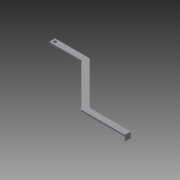
# Autodesk Inventor part: Z-PickupArm
Saved by Autodesk Inventor 2013 (Build 170138000, 138)
## iProperties
Created: 2014-01-22
Part Number: Z-PickupArm
Material: Generic
Document SubType Name: Modeling
Designer: Jarod
Density: 1 g/cm^3
Author: Jarod
Autodesk Inventor part; units mm, degrees
ref_plane "YZ Plane" through (0, 0, 0) normal (1, 0, 0) x (0, 1, 0)
ref_plane "XZ Plane" through (0, 0, 0) normal (0, 1, 0) x (-1, 0, 0)
ref_plane "XY Plane" through (0, 0, 0) normal (0, 0, 1) x (1, 0, 0)
sketch "Sketch1" plane through (0, 0, 0) normal (0, 1, 0) x (-1, 0, 0)
  line L0 (0, 0) -> (-139.7, 0)
  line L1 (-139.7, 0) -> (-139.7, 25.4)
  line L2 (-139.7, 25.4) -> (0, 25.4)
  line L3 (0, 25.4) -> (0, 0)
  line L4 (-139.7, 25.4) -> (-150.221, 0)
  line L5 (-139.7, 25.4) -> (-112.2072, 25.4) construction
  line L6 (-139.7, 25.4) -> (-157.6605, 7.4395)
  line L7 (-139.7, 25.4) -> (-114.3, 25.4) construction
  line L8 (-157.6605, 7.4395) -> (-150.221, 0)
  line L9 (-139.7, 25.4) -> (-157.6605, 7.4395)
  line L10 (-157.6605, 7.4395) -> (-337.2656, 187.0446)
  line L11 (-337.2656, 187.0446) -> (-319.3051, 205.0051)
  line L12 (-319.3051, 205.0051) -> (-139.7, 25.4)
  circle A0 centre (-12.7, 12.7) radius 6.35
  line L13 (-337.2656, 187.0446) -> (-515.0656, 187.0446)
  line L14 (-515.0656, 187.0446) -> (-515.0656, 212.4446)
  line L15 (-515.0656, 212.4446) -> (-337.2656, 212.4446)
  line L16 (-337.2656, 212.4446) -> (-337.2656, 187.0446)
  line L17 (-337.2656, 187.0446) -> (-326.7446, 212.4446)
  line L18 (-326.7446, 212.4446) -> (-337.2656, 212.4446)
  line L19 (-326.7446, 212.4446) -> (-319.3051, 205.0051)
  line L20 (-139.7, 0) -> (-150.221, 0)
  dimension "d0" = 139.7
  dimension "d1" = 25.4
  dimension "d2" = 112.5
  dimension "d3" = 25.4
  dimension "d4" = 135
  dimension "d5" = 254
  dimension "d6" = 12.7
  dimension "d7" = 177.8
  dimension "d8" = 25.4
  constraints: 42 end point, 7 parallel, 6 perpendicular, 4 horizontal, 2 equal length, 1 centre point
  measures "d0" distance of L1.end L2.end
  measures "d1" distance of L0.end L1.end
  measures "d2" angle of L4 L5
  measures "d3" distance of L1.end L6.end
  measures "d4" angle of L6 L7
  measures "d5" distance of L6.end L10.end
  measures "d6" diameter of A0
  measures "d7" distance of L14.end L15.end
  measures "d8" distance of L13.end L14.end
extrude "Extrusion1" add sketch "Sketch1" along normal blind 6.35
sketch "Sketch2" plane through (515.0656, 0, 212.4446) normal (1, 0, 0) x (0, 0, -1)
  line L0 (0, 6.35) -> (25.4, 6.35)
  line L1 (25.4, 6.35) -> (25.4, -19.05)
  line L2 (25.4, -19.05) -> (0, -19.05)
  line L3 (0, -19.05) -> (0, 6.35)
  point P0 (212.4446, 0)
  dimension "d11" = 25.4
  dimension "d12" = 25.4
  constraints: 8 end point, 2 parallel, 1 horizontal, 1 perpendicular
  measures "d11" distance of L1.end L2.end
  measures "d12" distance of L0.end L1.end
extrude "Extrusion2" add sketch "Sketch2" along normal blind 1.5875
body "Solid1"
